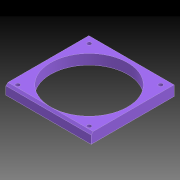
# Autodesk Inventor part: KB33-046-009 - Колпак лидара
Saved by Autodesk Inventor 2020 (Build 240168000, 168)
## iProperties
Created: 2021-08-10
Part Number: KB33-046-009 - Колпак лидара
Material: Типовые
Document SubType Name: Modeling
Designer: Петров Иван
Mass: 22.3263 g
Surface Area: 110.244 cm^2
Volume: 22.3263 cm^3
Density: 1 g/cm^3
Appearance: Фиолетовый
Author: Петров Иван
Autodesk Inventor part; units mm, degrees
ref_plane "YZ Plane" through (0, 0, 0) normal (1, 0, 0) x (0, 1, 0)
ref_plane "XZ Plane" through (0, 0, 0) normal (0, 1, 0) x (-1, 0, 0)
ref_plane "XY Plane" through (0, 0, 0) normal (0, 0, 1) x (1, 0, 0)
sketch "Эскиз1" plane through (0, 0, 0) normal (0, 1, 0) x (-1, 0, 0)
  circle A0 centre (35.3553, 35.3553) radius 2
  circle A1 centre (-35.3553, 35.3553) radius 2
  circle A2 centre (-35.3553, -35.3553) radius 2
  circle A3 centre (35.3553, -35.3553) radius 2
  line L0 (-40, 40) -> (40, 40)
  line L1 (40, 40) -> (40, -40)
  line L2 (40, -40) -> (-40, -40)
  line L3 (-40, -40) -> (-40, 40)
  line L4 (-40, 40) -> (40, -40) construction
  line L5 (40, 40) -> (-40, -40) construction
  point P0 (0, 0)
  dimension "d0" = 4
  dimension "d1" = 50
  dimension "d4" = 360
  dimension "d6" = 80
  dimension "d7" = 80
  constraints: 12 end point, 4 centre point, 2 midpoint, 2 parallel, 1 horizontal, 1 perpendicular, 1 point on line, 9 other
  measures "d0" diameter of A0
  measures "d1" distance of point (0, 0) A0.centre
  measures "d6" distance of L1.end L2.end
  measures "d7" distance of L0.end L1.end
extrude "Выдавливание1" add sketch "Эскиз1" along normal blind 10
sketch "Эскиз3" plane through (0, 10, 0) normal (0, 1, 0) x (1, 0, 0)
  circle A0 centre (0, 0) radius 37.5
  dimension "d16" = 75
  constraints: 1 centre point, 1 coincident
  measures "d16" diameter of A0
extrude "Выдавливание3" cut sketch "Эскиз3" against normal blind 10
thicken "Толщина1" operation add thickness 0.5 both sides no extend neighbours yes toward (0.9972038, 0, 0.0747301) faces at (37.3951, 3.3333, 2.8024)
move faces "Перенос1" translate (2, 0, 0) faces at (40, 6.6667, 13.3333)
move faces "Перенос2" translate (0, 0, -2) faces at (14.6667, 3.3333, -40)
move faces "Перенос3" translate (-2.25, 0, 0) faces at (-40, 3.3333, -14.6667)
sketch "Эскиз5" plane through (0, 0, 0) normal (0, -1, 0) x (1, 0, 0)
  circle A0 centre (35.3553, 35.3553) radius 2 projected
  line L0 (39.6855, 35.3553) -> (37.5204, 31.6053)
  line L1 (37.5204, 31.6053) -> (33.1903, 31.6053)
  line L2 (33.1903, 31.6053) -> (31.0252, 35.3553)
  line L3 (31.0252, 35.3553) -> (33.1903, 39.1053)
  line L4 (33.1903, 39.1053) -> (37.5204, 39.1053)
  line L5 (37.5204, 39.1053) -> (39.6855, 35.3553)
  point P0 (0, 0)
  dimension "d34" = 7.5
  constraints: 12 end point, 1 coincident, 13 other
  measures "d34" distance between parallel lines of L1 L4
extrude "Выдавливание5" cut sketch "Эскиз5" against normal blind 5
pattern_circular "Круговой массив2" count 4 over 360 about axis through (0, 10, 0) along (0, -1, 0) of "Выдавливание5"
chamfer "Фаска1" distance 2 angle 45 1 edges at (-0.125, 10, 40)
